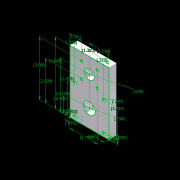
# Autodesk Inventor part: ytowerv1
Saved by Autodesk Inventor 2012 (Build 160160000, 160)
## iProperties
Created: 2011-09-19
Part Number: ytowerv1
Material: Default
Document SubType Name: Modeling
Designer: shane
Density: 1 g/cm^3
Author: shane
Autodesk Inventor part; units mm, degrees
ref_plane "YZ Plane" through (0, 0, 0) normal (1, 0, 0) x (0, 1, 0)
ref_plane "XZ Plane" through (0, 0, 0) normal (0, 1, 0) x (-1, 0, 0)
ref_plane "XY Plane" through (0, 0, 0) normal (0, 0, 1) x (1, 0, 0)
sketch "Sketch1" plane through (0, 0, 0) normal (0, 0, 1) x (1, 0, 0)
  line L0 (0, 0.3892) -> (63.5, 0.3892)
  line L1 (63.5, 0.3892) -> (63.5, 101.9892)
  line L2 (63.5, 101.9892) -> (0, 101.9892)
  line L3 (0, 101.9892) -> (0, 0.3892)
  point P0 (0, 0)
  dimension "d0" = 63.5
  dimension "d1" = 101.6
  constraints: 8 end point, 2 parallel, 1 horizontal, 1 perpendicular
  measures "d0" distance of L2.end L1.end
  measures "d1" distance of L1.end L0.end
extrude "Extrusion1" add sketch "Sketch1" along normal blind 12.7
hole "Hole15" at (8.128, 5.3422, 12.7) direction (0, 0, -1) diameter 5.08 end through all
hole "Hole16" at (55.372, 5.3422, 12.7) direction (0, 0, -1) diameter 5.08 end through all
hole "Hole17" at (8.128, 52.5862, 12.7) direction (0, 0, -1) diameter 5.08 end through all
hole "Hole18" at (55.372, 52.5862, 12.7) direction (0, 0, -1) diameter 5.08 end through all
hole "Hole19" at (31.75, 76.5892, 12.7) direction (0, 0, -1) diameter 15.9766 end through all
hole "Hole20" at (31.75, 28.9642, 12.7) direction (0, 0, -1) diameter 19.05 end through all
hole "Hole23" at (15.748, 0.3892, 6.35) direction (0, 1, 0) diameter 4.0386 depth 50.8 tip angle 118
hole "Hole24" at (47.752, 0.3892, 6.35) direction (0, 1, 0) diameter 4.0386 depth 50.8 tip angle 118
sketch "Font" plane through (0, 0, 12.7) normal (0, 0, 1) x (1, 0, 0)
  circle A0 centre (31.75, 28.9642) radius 9.525 projected
  circle A1 centre (31.75, 76.5892) radius 7.9883 projected
  circle A2 centre (55.372, 52.5862) radius 2.54 projected
  circle A3 centre (8.128, 52.5862) radius 2.54 projected
  circle A4 centre (55.372, 5.3422) radius 2.54 projected
  circle A5 centre (8.128, 5.3422) radius 2.54 projected
  line L0 (0, 0.3892) -> (0, 101.9892) projected
  line L1 (63.5, 0.3892) -> (0, 0.3892) projected
  line L2 (63.5, 101.9892) -> (63.5, 0.3892) projected
  line L3 (0, 101.9892) -> (63.5, 101.9892) projected
  point P0 (0, 0)
  dimension "d220" = 101.6
  dimension "d221" = 5.08
  dimension "d222" = 15.9766
  dimension "d223" = 19.05
  dimension "d224" = 8.128
  dimension "d225" = 4.953
  dimension "d226" = 28.575
  dimension "d227" = 76.2
  dimension "d228" = 8.128
  dimension "d229" = 4.953
  dimension "d230" = 52.197
  dimension "d231" = 52.197
  dimension "d237" = 31.75
  dimension "d238" = 31.75
  measures "d220" distance of L0.start L0.end
  measures "d221" diameter of A2
  measures "d222" diameter of A1
  measures "d223" diameter of A0
  measures "d224" distance from line of A3.centre L0
  measures "d225" distance from line of A5.centre L1
  measures "d226" distance from line of A0.centre L1
  measures "d227" distance from line of L1 A1.centre
  measures "d228" distance from line of A2.centre L2
  measures "d229" distance from line of L1 A4.centre
  measures "d230" distance from line of A3.centre L1
  measures "d231" distance from line of A2.centre L1
  measures "d237" distance from line of A1.centre L2
  measures "d238" distance from line of L2 A0.centre
sketch "Side" plane through (0, 0.3892, 0) normal (0, -1, 0) x (1, 0, 0)
  circle A0 centre (47.752, 6.35) radius 2.0193 projected
  circle A1 centre (15.748, 6.35) radius 2.0193 projected
  line L0 (63.5, 12.7) -> (0, 12.7) projected
  line L1 (0, 0) -> (0, 12.7) projected
  line L2 (0, 0) -> (63.5, 0) projected
  line L3 (63.5, 0) -> (63.5, 12.7) projected
  dimension "d232" = 15.748
  dimension "d233" = 12.7
  dimension "d234" = 15.748
  dimension "d235" = 6.35
  dimension "d236" = 6.35
  measures "d232" distance from line of L1 A1.centre
  measures "d233" distance of L2.end L0.start
  measures "d234" distance from line of A0.centre L3
  measures "d235" distance from line of L2 A1.centre
  measures "d236" distance from line of L2 A0.centre
hole "Hole25" at (19.05, 89.2892, 12.7) direction (0, 0, -1) diameter 3.937 end through all
hole "Hole26" at (19.05, 63.8892, 12.7) direction (0, 0, -1) diameter 3.937 end through all
hole "Hole27" at (44.45, 89.2892, 12.7) direction (0, 0, -1) diameter 3.937 end through all
hole "Hole28" at (44.45, 63.8892, 12.7) direction (0, 0, -1) diameter 3.937 end through all
sketch "Sketch5" plane through (0, 0, 12.7) normal (0, 0, 1) x (1, 0, 0)
  circle A0 centre (44.45, 63.8892) radius 1.9685 projected
  circle A1 centre (44.45, 89.2892) radius 1.9685 projected
  circle A2 centre (19.05, 63.8892) radius 1.9685 projected
  circle A3 centre (19.05, 89.2892) radius 1.9685 projected
  circle A4 centre (31.75, 28.9642) radius 9.525 projected
  circle A5 centre (31.75, 76.5892) radius 7.9883 projected
  circle A6 centre (55.372, 52.5862) radius 2.54 projected
  circle A7 centre (8.128, 52.5862) radius 2.54 projected
  circle A8 centre (55.372, 5.3422) radius 2.54 projected
  circle A9 centre (8.128, 5.3422) radius 2.54 projected
  line L0 (0, 0.3892) -> (0, 101.9892) projected
  line L1 (63.5, 0.3892) -> (0, 0.3892) projected
  line L2 (63.5, 101.9892) -> (63.5, 0.3892) projected
  line L3 (0, 101.9892) -> (63.5, 101.9892) projected
  point P0 (0, 0)
  dimension "d275" = 63.5
  dimension "d276" = 19.05
  dimension "d277" = 44.45
  dimension "d278" = 88.9
  measures "d275" distance from line of L1 A2.centre
  measures "d276" distance from line of L0 A3.centre
  measures "d277" distance from line of L0 A1.centre
  measures "d278" distance from line of L1 A3.centre
body "Solid1"
